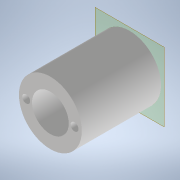
# Autodesk Inventor part: z axis motor cover
Saved by Autodesk Inventor 2021 (Build 250183000, 183)
## iProperties
Created: 2021-03-22
Part Number: z axis motor cover
Material: Generic
Document SubType Name: Modeling
Designer: ASUS
Density: 1 g/cm^3
Appearance: Default
Author: ASUS
Autodesk Inventor part; units mm, degrees
ref_plane "YZ Plane" through (0, 0, 0) normal (1, 0, 0) x (0, 1, 0)
ref_plane "XZ Plane" through (0, 0, 0) normal (0, 1, 0) x (-1, 0, 0)
ref_plane "XY Plane" through (0, 0, 0) normal (0, 0, 1) x (1, 0, 0)
ref_plane "Work Plane1" through (0, 0, -2) normal (0, 0, -1) x (-1, 0, 0)
sketch "Sketch1" plane through (0, 0, -2) normal (0, 0, -1) x (-1, 0, 0)
  circle A0 centre (0, 0) radius 18.5 construction
  circle A1 centre (0, 0) radius 19
  circle A2 centre (0, 0) radius 32.5
  circle A3 centre (25, 0) radius 3 construction
  circle A4 centre (-25, 0) radius 3 construction
  circle A5 centre (-25, 0) radius 4.1
  circle A6 centre (25, 0) radius 4.1
  dimension "d0" = 38
  dimension "d1" = 65
  dimension "d2" = 8.2
  dimension "d3" = 8.2
  constraints: 4 centre point, 3 coincident
  measures "d0" diameter of A1
  measures "d1" diameter of A2
  measures "d2" diameter of A5
  measures "d3" diameter of A6
ref_plane "Work Plane2" through (-93.3013, -86.3013, 80) normal (0, 0, -1) x (0, 1, 0)
extrude "Extrusion1" add sketch "Sketch1" against normal blind 80
sketch "Sketch2" plane through (0, 0, 78) normal (0, 0, 1) x (1, 0, 0)
  circle A0 centre (0, 0) radius 19 projected
  line L0 (-16.4545, -9.5) -> (-28.1458, -16.25)
  circle A1 centre (0, 0) radius 32.5 projected
  line L1 (-28.1458, -16.25) -> (0, 0) construction
  line L2 (0, 0) -> (0, -19) construction
  line L3 (16.4545, -9.5) -> (28.1458, -16.25)
  point P0 (0, 0)
  point P1 (16.4545, -9.5)
  dimension "d6" = 60
  constraints: 8 end point, 2 collinear, 2 point on circle, 2 symmetric about line, 1 vertical, 2 other
  measures "d6" angle of L2 L1
extrude "Extrusion2" cut sketch "Sketch2" against normal up to surface (80 mm away) contours A0 L3 A1 L0 picked at (0.7353, -27.8107)
sketch "Sketch3" plane through (0, 0, -2) normal (0, 0, -1) x (-1, 0, 0)
  line L0 (-16.4545, -9.5) -> (-28.1458, -16.25) projected
  arc A0 (16.4545, -9.5) -> (-16.4545, -9.5) centre (0, 0) ccw projected
  arc A1 (-16.4545, -9.5) -> (16.4545, -9.5) centre (0, 0) ccw
  arc A2 (28.1458, -16.25) -> (-28.1458, -16.25) centre (0, 0) ccw projected
  arc A3 (-28.1458, -16.25) -> (28.1458, -16.25) centre (0, 0) ccw
  line L1 (16.4545, -9.5) -> (28.1458, -16.25) projected
  constraints: 5 point on circle, 2 centre point, 2 coincident, 1 point on line
extrude "Extrusion3" add sketch "Sketch3" against normal blind 45 contours A1 L1 A3 L0
body "Solid1"
